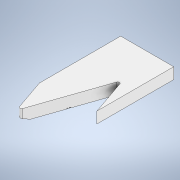
# Autodesk Inventor part: ketchenLightBracketV02-rightSide
Saved by Autodesk Inventor 2021.2 (Build 252289000, 289)
## iProperties
Created: 2021-01-10
Part Number: ketchenLightBracketV02-rightSide
Material: PC/ABS Plastic
Document SubType Name: Modeling
Designer: robst
Density: 0.357273 g/cm^3
Appearance: White
Author: robst
Autodesk Inventor part; units mm, degrees
ref_plane "YZ Plane" through (0, 0, 0) normal (1, 0, 0) x (0, 1, 0)
ref_plane "XZ Plane" through (0, 0, 0) normal (0, 1, 0) x (-1, 0, 0)
sketch "Sketch2" plane through (0, 0, 0) normal (0, 0, 1) x (1, 0, 0)
  line L0 (0, -33.7271) -> (0, 35.754) construction
  arc A0 (2.8938, 20.8) -> (0, 0) centre (76.2, 0) ccw
  line L1 (101.6, 0) -> (101.6, 20.8)
  line L2 (101.6, 20.8) -> (2.8938, 20.8)
  arc A1 (31.8545, 0) -> (7.0075, 0) centre (19.431, -7.3099) ccw
  line L3 (0, 0) -> (7.0075, 0)
  line L4 (31.8545, 0) -> (101.6, 0)
  dimension "d0" = 152.4
  dimension "d1" = 101.6
  dimension "d2" = 20.8
  dimension "d4" = 28.829
  dimension "d5" = 19.431
  constraints: 10 end point, 4 point on circle, 3 perpendicular, 2 centre point, 2 horizontal, 1 collinear, 1 tangent, 1 vertical
  measures "d0" diameter of A0
  measures "d1" distance of L3.start L1.start
  measures "d2" distance of L1.start L1.end
  measures "d4" diameter of A1
  measures "d5" horizontal distance of A1.centre L3.start
extrude "Extrusion1" add sketch "Sketch2" along normal mid plane 285.75
sketch "Sketch3" plane through (31.8545, 0, 142.875) normal (0, -1, 0) x (1, 0, 0)
  line L0 (69.7455, -285.75) -> (69.7455, 0) construction
  line L1 (0, -285.75) -> (0, 0) construction
  point P0 (-31.8545, -142.875)
  point P1 (58.3155, -12.7)
  dimension "d8" = 11.43
  measures "d8" distance from line of point (58.316, -12.7) L0
hole "Hole2" at (90.17, 0, 130.175) direction (0, 1, 0) diameter 3.302 depth 15.875 tip angle 118 thread size "8-32 UNC" class "2B" standard "ANSI Unified Screw Threads"
pattern_linear "Rectangular Pattern1" count 8 spacing 6.35 along (-1, 0, 0) of "Hole2"
sketch "SketchForText" plane through (31.8545, 0, 142.875) normal (0, -1, 0) x (1, 0, 0)
  line L0 (69.7455, 0) -> (69.7455, -285.75) construction
  line L1 (69.7455, -142.875) -> (0, -142.875) construction
  line L2 (0, -285.75) -> (0, 0) construction
  line L3 (54.5958, -146.685) -> (57.2202, -139.065)
  line L4 (57.2202, -139.065) -> (58.3132, -139.065)
  line L5 (58.3132, -139.065) -> (60.9376, -146.685)
  line L6 (60.9376, -146.685) -> (59.8508, -146.685)
  line L7 (59.8508, -146.685) -> (57.7389, -140.3556)
  line L8 (57.7389, -140.3556) -> (55.6271, -146.685)
  line L9 (55.6271, -146.685) -> (54.5958, -146.685)
  line L10 (51.2057, -141.9364) -> (54.0895, -141.9364)
  line L11 (54.0895, -141.9364) -> (54.0895, -142.8627)
  line L12 (54.0895, -142.8627) -> (51.2057, -142.8627)
  line L13 (51.2057, -142.8627) -> (51.2057, -141.9364)
  spline S0 degree 2 poles (45.4506, -142.875) (45.4506, -140.8249) (46.6424, -138.9044) (47.8836, -138.9044) knots 0 0 0 1 2 2 2
  spline S1 degree 2 poles (47.8836, -138.9044) (49.1433, -138.9044) (50.3227, -140.8619) (50.3227, -142.8688) knots 0 0 0 1 2 2 2
  spline S2 degree 2 poles (50.3227, -142.8688) (50.3227, -144.9313) (49.1309, -146.8394) (47.8836, -146.8394) knots 0 0 0 1 2 2 2
  spline S3 degree 2 poles (47.8836, -146.8394) (46.63, -146.8394) (45.4506, -144.8634) (45.4506, -142.875) knots 0 0 0 1 2 2 2
  spline S4 degree 2 poles (46.7597, -140.5532) (46.6115, -140.9299) (46.488, -142.0908) (46.488, -142.875) knots 0 0 0 1 2 2 2
  spline S5 degree 2 poles (46.488, -142.875) (46.488, -143.6592) (46.6115, -144.814) (46.7659, -145.203) knots 0 0 0 1 2 2 2
  spline S6 degree 2 poles (46.7659, -145.203) (46.9203, -145.592) (47.4575, -145.9934) (47.8836, -145.9934) knots 0 0 0 1 2 2 2
  spline S7 degree 2 poles (47.8836, -145.9934) (48.3096, -145.9934) (48.8592, -145.592) (49.0198, -145.1906) knots 0 0 0 1 2 2 2
  spline S8 degree 2 poles (49.0198, -145.1906) (49.1741, -144.8016) (49.2853, -143.616) (49.2853, -142.8688) knots 0 0 0 1 2 2 2
  spline S9 degree 2 poles (49.2853, -142.8688) (49.2853, -142.0661) (49.1865, -140.9916) (49.0259, -140.5717) knots 0 0 0 1 2 2 2
  spline S10 degree 2 poles (49.0259, -140.5717) (48.8777, -140.1765) (48.3282, -139.7504) (47.8836, -139.7504) knots 0 0 0 1 2 2 2
  spline S11 degree 2 poles (47.8836, -139.7504) (47.4637, -139.7504) (46.9141, -140.1518) (46.7597, -140.5532) knots 0 0 0 1 2 2 2
  line L14 (39.7757, -139.065) -> (44.4749, -139.065)
  line L15 (44.4749, -139.065) -> (44.4749, -140.1456)
  spline S12 degree 2 poles (44.4749, -140.1456) (43.9686, -140.6211) (43.067, -141.5041) (42.6348, -141.9796) knots 0 0 0 1 2 2 2
  spline S13 degree 2 poles (42.6348, -141.9796) (41.7641, -142.9368) (41.1281, -144.0853) (41.1281, -144.6966) knots 0 0 0 1 2 2 2
  spline S14 degree 2 poles (41.1281, -144.6966) (41.1281, -145.0177) (41.3257, -145.4994) (41.5047, -145.6538) knots 0 0 0 1 2 2 2
  spline S15 degree 2 poles (41.5047, -145.6538) (41.6838, -145.8081) (42.1531, -145.9625) (42.4372, -145.9625) knots 0 0 0 1 2 2 2
  spline S16 degree 2 poles (42.4372, -145.9625) (42.7089, -145.9625) (43.2646, -145.8267) (43.5178, -145.7217) knots 0 0 0 1 2 2 2
  spline S17 degree 2 poles (43.5178, -145.7217) (43.7339, -145.6352) (44.1353, -145.3882) (44.2588, -145.3018) knots 0 0 0 1 2 2 2
  line L16 (44.2588, -145.3018) -> (44.3144, -145.3018)
  line L17 (44.3144, -145.3018) -> (44.3144, -146.3886)
  spline S18 degree 2 poles (44.3144, -146.3886) (43.9995, -146.543) (42.8694, -146.8456) (42.3631, -146.8456) knots 0 0 0 1 2 2 2
  spline S19 degree 2 poles (42.3631, -146.8456) (41.2948, -146.8456) (40.0907, -145.7155) (40.0907, -144.7522) knots 0 0 0 1 2 2 2
  spline S20 degree 2 poles (40.0907, -144.7522) (40.0907, -144.3014) (40.3006, -143.5481) (40.4859, -143.227) knots 0 0 0 1 2 2 2
  spline S21 degree 2 poles (40.4859, -143.227) (40.6711, -142.8935) (41.2083, -142.239) (41.5047, -141.924) knots 0 0 0 1 2 2 2
  spline S22 degree 2 poles (41.5047, -141.924) (41.9864, -141.3992) (43.1658, -140.2753) (43.5178, -139.948) knots 0 0 0 1 2 2 2
  line L18 (43.5178, -139.948) -> (39.7757, -139.948)
  line L19 (39.7757, -139.948) -> (39.7757, -139.065)
  spline S23 degree 2 poles (30.4514, -144.3879) (30.4514, -143.8939) (30.8034, -143.0047) (31.1183, -142.6959) knots 0 0 0 1 2 2 2
  spline S24 degree 2 poles (31.1183, -142.6959) (31.5135, -142.3069) (32.5818, -141.9055) (33.3969, -141.9055) knots 0 0 0 1 2 2 2
  line L20 (33.3969, -141.9055) -> (34.2552, -141.9055)
  line L21 (34.2552, -141.9055) -> (34.2552, -139.065)
  line L22 (34.2552, -139.065) -> (35.268, -139.065)
  line L23 (35.268, -139.065) -> (35.268, -146.685)
  line L24 (35.268, -146.685) -> (33.3537, -146.685)
  spline S25 degree 2 poles (33.3537, -146.685) (32.6744, -146.685) (31.7235, -146.4627) (31.3592, -146.2095) knots 0 0 0 1 2 2 2
  spline S26 degree 2 poles (31.3592, -146.2095) (30.9331, -145.9193) (30.4514, -145.0239) (30.4514, -144.3879) knots 0 0 0 1 2 2 2
  spline S27 degree 2 poles (31.5074, -144.357) (31.5074, -144.7522) (31.7791, -145.3327) (32.0569, -145.5179) knots 0 0 0 1 2 2 2
  spline S28 degree 2 poles (32.0569, -145.5179) (32.2978, -145.6785) (32.94, -145.8081) (33.4154, -145.8081) knots 0 0 0 1 2 2 2
  line L25 (33.4154, -145.8081) -> (34.2552, -145.8081)
  line L26 (34.2552, -145.8081) -> (34.2552, -142.77)
  line L27 (34.2552, -142.77) -> (33.5636, -142.77)
  spline S29 degree 2 poles (33.5636, -142.77) (32.9461, -142.77) (32.1866, -142.9676) (31.9396, -143.227) knots 0 0 0 1 2 2 2
  spline S30 degree 2 poles (31.9396, -143.227) (31.7111, -143.4555) (31.5074, -143.9927) (31.5074, -144.357) knots 0 0 0 1 2 2 2
  line L28 (23.9615, -146.685) -> (26.5858, -139.065)
  line L29 (26.5858, -139.065) -> (27.6788, -139.065)
  line L30 (27.6788, -139.065) -> (30.3032, -146.685)
  line L31 (30.3032, -146.685) -> (29.2164, -146.685)
  line L32 (29.2164, -146.685) -> (27.1045, -140.3556)
  line L33 (27.1045, -140.3556) -> (24.9927, -146.685)
  line L34 (24.9927, -146.685) -> (23.9615, -146.685)
  line L35 (20.5714, -141.9364) -> (23.4551, -141.9364)
  line L36 (23.4551, -141.9364) -> (23.4551, -142.8627)
  line L37 (23.4551, -142.8627) -> (20.5714, -142.8627)
  line L38 (20.5714, -142.8627) -> (20.5714, -141.9364)
  spline S31 degree 2 poles (14.8162, -142.875) (14.8162, -140.8249) (16.008, -138.9044) (17.2492, -138.9044) knots 0 0 0 1 2 2 2
  spline S32 degree 2 poles (17.2492, -138.9044) (18.5089, -138.9044) (19.6883, -140.8619) (19.6883, -142.8688) knots 0 0 0 1 2 2 2
  spline S33 degree 2 poles (19.6883, -142.8688) (19.6883, -144.9313) (18.4965, -146.8394) (17.2492, -146.8394) knots 0 0 0 1 2 2 2
  spline S34 degree 2 poles (17.2492, -146.8394) (15.9957, -146.8394) (14.8162, -144.8634) (14.8162, -142.875) knots 0 0 0 1 2 2 2
  spline S35 degree 2 poles (16.1253, -140.5532) (15.9771, -140.9299) (15.8536, -142.0908) (15.8536, -142.875) knots 0 0 0 1 2 2 2
  spline S36 degree 2 poles (15.8536, -142.875) (15.8536, -143.6592) (15.9771, -144.814) (16.1315, -145.203) knots 0 0 0 1 2 2 2
  spline S37 degree 2 poles (16.1315, -145.203) (16.2859, -145.592) (16.8231, -145.9934) (17.2492, -145.9934) knots 0 0 0 1 2 2 2
  spline S38 degree 2 poles (17.2492, -145.9934) (17.6753, -145.9934) (18.2248, -145.592) (18.3854, -145.1906) knots 0 0 0 1 2 2 2
  spline S39 degree 2 poles (18.3854, -145.1906) (18.5398, -144.8016) (18.6509, -143.616) (18.6509, -142.8688) knots 0 0 0 1 2 2 2
  spline S40 degree 2 poles (18.6509, -142.8688) (18.6509, -142.0661) (18.5521, -140.9916) (18.3916, -140.5717) knots 0 0 0 1 2 2 2
  spline S41 degree 2 poles (18.3916, -140.5717) (18.2434, -140.1765) (17.6938, -139.7504) (17.2492, -139.7504) knots 0 0 0 1 2 2 2
  spline S42 degree 2 poles (17.2492, -139.7504) (16.8293, -139.7504) (16.2797, -140.1518) (16.1253, -140.5532) knots 0 0 0 1 2 2 2
  spline S43 degree 2 poles (9.024, -141.535) (9.024, -140.9484) (9.4131, -139.9542) (9.7403, -139.6208) knots 0 0 0 1 2 2 2
  spline S44 degree 2 poles (9.7403, -139.6208) (10.08, -139.2688) (10.9321, -138.9044) (11.4446, -138.9044) knots 0 0 0 1 2 2 2
  spline S45 degree 2 poles (11.4446, -138.9044) (11.9572, -138.9044) (12.8032, -139.2503) (13.1243, -139.5961) knots 0 0 0 1 2 2 2
  spline S46 degree 2 poles (13.1243, -139.5961) (13.5195, -140.0098) (13.9641, -141.3992) (13.9641, -142.4119) knots 0 0 0 1 2 2 2
  spline S47 degree 2 poles (13.9641, -142.4119) (13.9641, -143.4061) (13.5565, -145.0054) (13.1304, -145.5982) knots 0 0 0 1 2 2 2
  spline S48 degree 2 poles (13.1304, -145.5982) (12.7167, -146.1786) (11.4076, -146.827) (10.5493, -146.827) knots 0 0 0 1 2 2 2
  spline S49 degree 2 poles (10.5493, -146.827) (10.2961, -146.827) (9.8515, -146.7776) (9.6848, -146.7221) knots 0 0 0 1 2 2 2
  line L39 (9.6848, -146.7221) -> (9.6848, -145.7402)
  line L40 (9.6848, -145.7402) -> (9.728, -145.7402)
  spline S50 degree 2 poles (9.728, -145.7402) (9.87, -145.8143) (10.3887, -145.944) (10.6851, -145.944) knots 0 0 0 1 2 2 2
  spline S51 degree 2 poles (10.6851, -145.944) (11.6361, -145.944) (12.8032, -144.6596) (12.9143, -143.3999) knots 0 0 0 1 2 2 2
  spline S52 degree 2 poles (12.9143, -143.3999) (12.55, -143.6531) (11.7843, -143.9309) (11.3273, -143.9309) knots 0 0 0 1 2 2 2
  spline S53 degree 2 poles (11.3273, -143.9309) (10.8827, -143.9309) (10.2158, -143.7519) (9.8515, -143.4802) knots 0 0 0 1 2 2 2
  spline S54 degree 2 poles (9.8515, -143.4802) (9.4316, -143.1652) (9.024, -142.1896) (9.024, -141.535) knots 0 0 0 1 2 2 2
  spline S55 degree 2 poles (10.0614, -141.4918) (10.0614, -141.9611) (10.3084, -142.5971) (10.5801, -142.8194) knots 0 0 0 1 2 2 2
  spline S56 degree 2 poles (10.5801, -142.8194) (10.7839, -142.98) (11.2903, -143.085) (11.5558, -143.085) knots 0 0 0 1 2 2 2
  spline S57 degree 2 poles (11.5558, -143.085) (11.9139, -143.085) (12.587, -142.8688) (12.9143, -142.665) knots 0 0 0 1 2 2 2
  spline S58 degree 2 poles (12.9143, -142.665) (12.9205, -142.5539) (12.9328, -142.3439) (12.9328, -142.1834) knots 0 0 0 1 2 2 2
  spline S59 degree 2 poles (12.9328, -142.1834) (12.9328, -141.393) (12.6241, -140.4235) (12.3894, -140.1703) knots 0 0 0 1 2 2 2
  spline S60 degree 2 poles (12.3894, -140.1703) (12.1733, -139.9295) (11.704, -139.7381) (11.4385, -139.7381) knots 0 0 0 1 2 2 2
  spline S61 degree 2 poles (11.4385, -139.7381) (10.821, -139.7381) (10.0614, -140.6149) (10.0614, -141.4918) knots 0 0 0 1 2 2 2
  point P0 (-31.8545, -142.875)
  constraints: 2 end point, 2 midpoint, 1 horizontal
extrude "ExtrusionForText" cut sketch "SketchForText" against normal blind 1.27
ref_plane "Work Plane1" through (0, 0, 92.075) normal (0, 0, 1) x (1, 0, 0)
mirror "MirrorHoles" about plane through (0, 0, 0) normal (0, 0, 1) of "Hole2", "Rectangular Pattern1"
sketch "SketchForSplittingPart" plane through (2.8938, 20.8, 142.875) normal (0, 1, 0) x (1, 0, 0)
  line L0 (-2.8938, 285.75) -> (-2.8938, 0) projected
  line L1 (0, 285.75) -> (98.7062, 285.75) projected
  line L2 (98.7062, 285.75) -> (98.7062, 0) projected
  line L3 (98.7062, 0) -> (0, 0) projected
  line L4 (-2.8938, 0) -> (98.7062, 0)
  line L5 (98.7062, 0) -> (98.7062, 285.75)
  line L6 (98.7062, 285.75) -> (-2.8938, 285.75)
  line L7 (-2.8938, 285.75) -> (-2.8938, 0)
  line L8 (98.7062, 142.875) -> (-2.8938, 142.875) construction
  line L9 (47.9062, 142.875) -> (47.9062, 285.75) construction
  line L10 (98.7062, 142.875) -> (76.3082, 207.9084)
  line L11 (70.3043, 207.9084) -> (47.9062, 142.875)
  line L12 (47.9062, 142.875) -> (25.5082, 77.8416)
  line L13 (56.6395, 139.065) -> (59.2639, 146.685) projected
  line L14 (19.5043, 77.8416) -> (-2.8938, 142.875)
  arc A0 (76.3082, 207.9084) -> (70.3043, 207.9084) centre (73.3062, 206.8745) ccw
  arc A1 (19.5043, 77.8416) -> (25.5082, 77.8416) centre (22.5062, 78.8755) ccw
  point P0 (-2.8938, 142.875)
  dimension "d30" = 3.175
  dimension "d31" = 3.175
  constraints: 20 end point, 4 parallel, 4 point on circle, 4 tangent, 3 equal length, 3 midpoint, 2 centre point, 2 perpendicular, 1 horizontal, 1 point on line
  measures "d30" radius of A0
  measures "d31" radius of A1
extrude "Extrusion3" cut sketch "SketchForSplittingPart" against normal through all contours L14 A1 L12 L11 A0 L10 L2 L3 L4 L0
equation "\"d0\" = 2 * radiusOfCurvatureForWall"
equation "\"d1\" = distanceFromWall"
equation "\"d2\" = thickness"
equation "\"d4\" = dometicDiameter"
equation "\"d5\" = dometicCenterDistanceFromWall"
equation "\"d6\" = width"
equation "\"d8\" = startingHole"
equation "\"thickness\" = 20.8"
equation "\"distanceFromWall\" = 101.6"
equation "\"radiusOfCurvatureForWall\" = 76.2"
equation "\"dometicDiameter\" = 28.829"
equation "\"dometicCenterDistanceFromWall\" = 19.431"
equation "\"startingHole\" = 11.43"
equation "\"width\" = 285.75"
body "Solid1"
